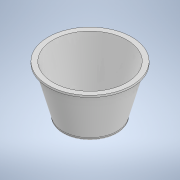
# Autodesk Inventor part: pingPongHolder 1-13
Saved by Autodesk Inventor 2020 (Build 240168000, 168)
## iProperties
Created: 2020-01-14
Part Number: pingPongHolder 1-13
Material: Generic
Document SubType Name: Modeling
Designer: akend
Density: 1 g/cm^3
Appearance: Default
Author: akend
## iProperties of the stored document _3DPrint.ipt
Created: 2020-01-14
Part Number: _3DPrint
Material: Generic
Document SubType Name: Modeling
Designer: akend
Density: 1 g/cm^3
Appearance: Default
Author: akend
Autodesk Inventor part; units mm, degrees
ref_plane "YZ Plane" through (0, 0, 0) normal (1, 0, 0) x (0, 1, 0)
ref_plane "XZ Plane" through (0, 0, 0) normal (0, 1, 0) x (-1, 0, 0)
ref_plane "XY Plane" through (0, 0, 0) normal (0, 0, 1) x (1, 0, 0)
sketch "Sketch1" plane through (0, 0, 0) normal (1, 0, 0) x (0, 1, 0)
  line L0 (0, 0) -> (0, 25)
  line L1 (0, 25) -> (48.2963, 37.941)
  line L2 (48.2963, 37.941) -> (48.2963, 42.941)
  line L3 (48.2963, 42.941) -> (46.2963, 42.941)
  line L4 (0, 25) -> (0, 28)
  line L5 (0, 28) -> (46.2963, 40.4051)
  line L6 (0, 28) -> (-3, 28)
  line L7 (-3, 28) -> (-3, 0)
  line L8 (-3, 0) -> (0, 0)
  line L9 (0, 0) -> (0, 28)
  line L10 (46.2963, 42.941) -> (46.2963, 40.4051)
  line L11 (0, 28) -> (0, 25)
  line L12 (0, 25) -> (48.2963, 37.941)
  line L13 (48.2963, 37.941) -> (48.2963, 42.941)
  line L14 (48.2963, 42.941) -> (46.2963, 42.941)
  line L15 (46.2963, 42.941) -> (46.2963, 40.4051)
  line L16 (46.2963, 40.4051) -> (0, 28)
  line L17 (0, 28) -> (0, 25)
  dimension "d0" = 25
  dimension "d1" = 50
  dimension "d2" = 105
  dimension "d3" = 5
  dimension "d4" = 2
  dimension "d5" = 3
  dimension "d6" = 105
  dimension "d7" = 3
  constraints: 36 end point, 4 collinear, 4 vertical, 3 parallel, 3 perpendicular, 1 horizontal
  measures "d0" distance of L0.start L0.end
  measures "d1" distance of L0.end L1.end
  measures "d2" angle of L0 L1
  measures "d3" distance of L1.end L2.end
  measures "d4" distance of L2.end L3.end
  measures "d5" distance of L0.end L4.end
  measures "d6" angle of L4 L5
  measures "d7" distance of L8.end L7.end
sketch "Sketch2" plane through (0, 0, 0) normal (1, 0, 0) x (0, 1, 0)
  line L0 (0, 0) -> (3.3899, 0)
  constraints: 2 end point, 1 horizontal
revolve "Revolution1" add sketch "Sketch1" angle 360 about axis through (0, 0, 0) along (0, 1, 0)
fillet "Fillet1" radius 2 1 edges at (0, -3, -28)
body "Solid1"
